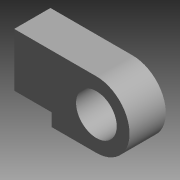
# Autodesk Inventor part: Lower Arm Bracket
Saved by Autodesk Inventor 2014 SP1 (Build 180222100, 222)
## iProperties
Created: 2013-12-29
Part Number: Lower Arm Bracket
Material: Generic
Document SubType Name: Modeling
Designer: tom
Density: 1 g/cm^3
Appearance: Default
Author: tom
Autodesk Inventor part; units mm, degrees
ref_plane "YZ Plane" through (0, 0, 0) normal (1, 0, 0) x (0, 1, 0)
ref_plane "XZ Plane" through (0, 0, 0) normal (0, 1, 0) x (-1, 0, 0)
ref_plane "XY Plane" through (0, 0, 0) normal (0, 0, 1) x (1, 0, 0)
sketch "Sketch1" plane through (0, 0, 0) normal (0, 0, 1) x (1, 0, 0)
  line L0 (0, 0) -> (0, -3.175)
  line L1 (0, -3.175) -> (5.16, -3.175)
  line L2 (0, 0) -> (0, 5.175)
  line L3 (0, 5.175) -> (12.66, 5.175)
  arc A0 (12.66, -5.175) -> (12.66, 5.175) centre (12.66, 0) ccw
  line L4 (12.66, -5.175) -> (5.66, -5.175)
  line L5 (5.66, -5.175) -> (5.66, -3.675)
  circle A1 centre (12.66, 0) radius 3.175
  arc A2 (5.66, -3.675) -> (5.16, -3.175) centre (5.66, -3.175) ccw
  dimension "d3" = 5.175
  dimension "d4" = 6.35
  dimension "d7" = 7
  dimension "d9" = 2
  dimension "d10" = 5.66
  dimension "d11" = 1
  dimension "d12" = 5.66
  constraints: 12 end point, 4 point on circle, 3 centre point, 3 perpendicular, 1 coincident, 1 parallel, 1 tangent, 1 vertical
  measures "d3" distance of L0.start L2.end
  measures "d4" diameter of A1
  measures "d7" distance from line of L5 A0.centre
  measures "d9" radial gap between concentric circles of A0 A1
  measures "d10" distance between parallel lines of L5 L0
  measures "d11" diameter of A2
  measures "d12" distance of L0.end A2.centre
extrude "Extrusion1" add sketch "Sketch1" along normal blind 5.66
body "Solid1"
